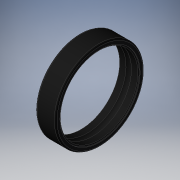
# Autodesk Inventor part: 6007DDU Outer ring
Saved by Autodesk Inventor 2023 (Build 270158000, 158)
## iProperties
Created: 2023-07-20
Part Number: 6007DDU Outer ring
Material: Generic
Catalog Web Link: www.cadenas.de
Description: contact_sealed_type_dd_ddu_OR-NSK
Vendor: NSK_RB
Document SubType Name: Modeling
Designer: psAdmin
Manufacturer: NSK_RB
Mass: 9.53823 g
Surface Area: 64.3529 cm^2
Volume: 9.53823 cm^3
Density: 1 g/cm^3
Appearance: PSOLRGB-128-128-128
Category: PARTsolutions
Company: NSK_RB
PSOL_IDENT_0: {$CADENAS_DATA/23d-libs/nsk_rb/roller_bearings/deep_groove_bb/single_row_dgbb/contact_sealed_type_dd
PSOL_IDENT_1: _ddu_1_or.prj},201 {VTYP=3D},{NB=6007DDU Outer ring},{LINA=6007DDU Outer ring},{NN=contact_sealed_ty
PSOL_IDENT_2: pe_dd_ddu_OR},{DATE=15.09.2022 00:32:48},{GEOMDATE=08.08.2022 08:01:00},{VERSION=},{LINEID=1980},{WB
PSOL_IDENT_3: VAR=},{WBNUMERIC=}  {NB=6007DDU Outer ring},{LINA=6007DDU Outer ring},{KT=DUMMY},{IDNR=21},{STAN=Sta
PSOL_IDENT_4: ndard},{ORDER=6007DDU},{SD=35},{X=35},{DI1=43.50},{DI2=41.6},{SDE1=54.10},{SDE2=56.00},{D=62},{DD=62
PSOL_IDENT_5: },{B=14},{R=1.0},{CR1=16000},{COR1=10300},{CR2=1630},{COR2=1050},{FO=14.8},{LG=6700},{A=2.08},{BB=1.
PSOL_IDENT_6: 90},{DD1=59.61},{RO=0.60},{RN=0.5},{DD2=67.7},{F=1.70},{DAM1=40.0},{DA1=41.5},{DA2=57.0},{RA=1.0},{D
PSOL_IDENT_7: X=68.5},{CY=3.4},{MASS=0.151},{SC=1},{DIST=2.533}
NB: 6007DDU Outer ring
NN: contact_sealed_type_dd_ddu_OR
NT: NSK
NBSYN: $ORDER. Outer ring
LINA: 6007DDU Outer ring
CATALOG: NSK Rolling Bearing
IDNR: 21
STAN: Standard
ORDER: 6007DDU
SD: 35
X: 35
DI1: 43.5
DI2: 41.6
SDE1: 54.1
SDE2: 56
D: 62
DD: 62
B: 14
R: 1
CR1: 16000
COR1: 10300
CR2: 1630
COR2: 1050
FO: 14.8
LG: 6700
A: 2.08
BB: 1.9
DD1: 59.61
RO: 0.6
RN: 0.5
DD2: 67.7
F: 1.7
DAM1: 40
DA1: 41.5
DA2: 57
RA: 1
DX: 68.5
CY: 3.4
MASS: 0.151
SC: 1
SUPPLIER: NSK_RB
ARTICLENO: 6007DDU Outer ring
BOMINFO: 6007DDU Outer ring
CREATOR: CADENAS GmbH
Title: 6007DDU Outer ring
Author: Cadenas PARTsolutions
Comments: NSK
Autodesk Inventor part; units mm, degrees
sketch "Sketch_1" plane through (0, 0, 0) normal (0, 0, 1) x (1, 0, 0)
  line L0 (14, 0) -> (0, 0)
  line L1 (0, 28) -> (0.644, 28)
  line L2 (0.644, 28) -> (0.644, 27.05)
  line L3 (0.644, 27.05) -> (5.1157, 27.05)
  arc A0 (8.8843, 27.05) -> (5.1157, 27.05) centre (7, 24.25) ccw
  line L4 (8.8843, 27.05) -> (13.356, 27.05)
  line L5 (13.356, 27.05) -> (13.356, 28)
  line L6 (13.356, 28) -> (14, 28)
  line L7 (14, 28) -> (14, 30)
  arc A1 (14, 30) -> (13, 31) centre (13, 30) ccw
  line L8 (13, 31) -> (1, 31)
  arc A2 (1, 31) -> (0, 30) centre (1, 30) ccw
  line L9 (0, 30) -> (0, 28)
  constraints: 20 end point, 6 point on circle, 3 centre point
revolve "Revolution1" add sketch "Sketch_1" angle 360 about axis through (14, 0, 0) along (1, 0, 0)
ref_plane "ip_cst_1_or_1_XY" through (0, 0, 0) normal (1, 0, 0) x (0, 0, -1)
ref_plane "ip_cst_1_or_1_YZ" through (0, 0, 0) normal (0, 0, -1) x (0, 1, 0)
ref_plane "ip_cst_1_or_1_ZX" through (0, 0, 0) normal (0, 1, 0) x (1, 0, 0)
ref_plane "ip_cst_1_or_2_XY" through (0, 0, 0) normal (-1, 0, 0) x (0, 0, -1)
ref_plane "ip_cst_1_or_2_YZ" through (0, 0, 0) normal (0, 0, -1) x (0, -1, 0)
ref_plane "ip_cst_1_or_2_ZX" through (0, 0, 0) normal (0, -1, 0) x (-1, 0, 0)
ref_plane "ip_cst_1_or_3_XY" through (0.644, 0, 0) normal (1, 0, 0) x (0, 0, -1)
ref_plane "ip_cst_1_or_3_YZ" through (0.644, 0, 0) normal (0, 0, -1) x (0, 1, 0)
ref_plane "ip_cst_1_or_3_ZX" through (0.644, 0, 0) normal (0, 1, 0) x (1, 0, 0)
ref_plane "ip_cst_1_or_4_XY" through (13.356, 0, 0) normal (-1, 0, 0) x (0, 0, -1)
ref_plane "ip_cst_1_or_4_YZ" through (13.356, 0, 0) normal (0, 0, -1) x (0, -1, 0)
ref_plane "ip_cst_1_or_4_ZX" through (13.356, 0, 0) normal (0, -1, 0) x (-1, 0, 0)
body "Solid1"
